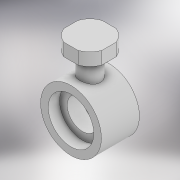
# Autodesk Inventor part: Sholder
Saved by Autodesk Inventor 2022 (Build 260153000, 153)
## iProperties
Created: 2022-02-25
Part Number: Sholder
Material: Generic
Document SubType Name: Modeling
Designer: joshw
Density: 1 g/cm^3
Appearance: Default
Author: joshw
Autodesk Inventor part; units mm, degrees
ref_plane "YZ Plane" through (0, 0, 0) normal (1, 0, 0) x (0, 1, 0)
ref_plane "XZ Plane" through (0, 0, 0) normal (0, 1, 0) x (-1, 0, 0)
ref_plane "XY Plane" through (0, 0, 0) normal (0, 0, 1) x (1, 0, 0)
sketch "Sketch1" plane through (0, 0, 0) normal (0, 0, 1) x (1, 0, 0)
  point P0 (0, 0)
sketch "Sketch2" plane through (0, 0, 0) normal (0, 0, 1) x (1, 0, 0)
  line L0 (12.1777, -1.5396) -> (4.6777, -1.5396) construction
  line L1 (4.6777, -1.5396) -> (4.6777, -5.5396) construction
  line L2 (4.6777, -5.5396) -> (12.1777, -5.5396) construction
  line L3 (12.1777, -5.5396) -> (12.1777, -1.5396) construction
  line L4 (8.4277, -4.7896) -> (12.4277, -4.7896)
  line L5 (12.4277, -4.7896) -> (12.4277, -2.2896)
  line L6 (12.4277, -2.2896) -> (8.4277, -2.2896)
  line L7 (8.4277, -2.2896) -> (8.4277, -4.7896)
  line L8 (8.4277, -2.2896) -> (8.4277, -8.9787)
  line L9 (8.4277, -8.9787) -> (10.4777, -8.9787)
  line L10 (10.4777, -8.9787) -> (10.4777, -4.7896)
  line L11 (9.1419, -2.2896) -> (9.1419, -1.5396) construction
  line L12 (9.1419, -4.7896) -> (9.1419, -5.5396) construction
  point P0 (0, 0)
  dimension "d0" = 7.5
  dimension "d1" = 4
  dimension "d2" = 8
  dimension "d3" = 2.5
  dimension "d4" = 4.1
  dimension "d6" = 0.75
  constraints: 26 end point, 6 perpendicular, 5 point on line, 4 parallel, 2 horizontal, 1 collinear, 1 vertical
  measures "d0" distance of L2.end L2.start
  measures "d1" distance of L2.start L1.start
  measures "d2" diameter of L5 L7
  measures "d3" distance between parallel lines of L6 L4
  measures "d4" diameter of L10 L7
  measures "d6" distance of L12.start L12.end
revolve "Revolution1" add sketch "Sketch2" angle 360 about axis through (8.4277, -2.2896, 0) along (0, -1, 0)
sketch "Sketch3" plane through (8.4277, -8.9787, 0) normal (0, -1, 0) x (1, 0, 0)
  line L0 (6, 3.75) -> (-6, 3.75)
  line L1 (-6, 3.75) -> (-6, -3.75)
  line L2 (-6, -3.75) -> (6, -3.75)
  line L3 (6, -3.75) -> (6, 3.75)
  line L4 (6, 3.75) -> (-6, -3.75) construction
  line L5 (-6, 3.75) -> (6, -3.75) construction
  circle A0 centre (0, 0) radius 2.05 projected
  point P0 (-8.4277, 0)
  point P1 (0, 0)
  dimension "d7" = 12
  dimension "d8" = 7.5
  constraints: 12 end point, 3 midpoint, 2 coincident, 2 parallel, 1 horizontal, 1 perpendicular
  measures "d7" distance of L2.end L1.end
  measures "d8" distance of L1.end L0.end
extrude "Extrusion1" add sketch "Sketch3" along normal blind 12 contours L3 L2 L1 L0 | A0
sketch "Sketch4" plane through (14.4277, -8.9787, -3.75) normal (0, 0, -1) x (-1, 0, 0)
  line L0 (12, 0) -> (0, 0) projected
  line L1 (0, 0) -> (0, -12) projected
  line L2 (12, -12) -> (0, -12) projected
  line L3 (12, 0) -> (12, -12) projected
  circle A0 centre (6, -6) radius 6
  point P0 (14.4277, 8.9787)
  point P1 (0, -6)
  point P2 (6, 0)
  point P3 (12, -6)
  point P4 (6, -12)
  constraints: 3 tangent, 1 centre point
extrude "Extrusion2" cut sketch "Sketch4" against normal blind 12 contours L3 A0 L0 | A0 L1 L0 | L3 L2 A0 | A0 L2 L1
sketch "Sketch6" plane through (0, 0, 0) normal (0, 0, 1) x (1, 0, 0)
  circle A0 centre (8.4277, -14.9787) radius 6 projected
  circle A1 centre (8.4277, -14.9787) radius 3
  point P0 (0, 0)
  dimension "d13" = 6
  constraints: 1 centre point, 1 coincident
  measures "d13" diameter of A1
extrude "Extrusion3" cut sketch "Sketch6" along normal mid plane 3 contours A1
sketch "Sketch7" plane through (8.4277, -14.9787, 1.5) normal (0, 0, -1) x (-1, 0, 0)
  circle A0 centre (0, 0) radius 3 projected
  circle A1 centre (0, 0) radius 4.5
  point P0 (8.4277, 14.9787)
  dimension "d16" = 9
  constraints: 1 centre point, 1 coincident
  measures "d16" diameter of A1
extrude "Extrusion4" cut sketch "Sketch7" against normal blind 8.25 contours A0 | A1
sketch "Sketch8" plane through (8.4277, -14.9787, -1.5) normal (0, 0, 1) x (1, 0, 0)
  circle A0 centre (0, 0) radius 4.5 projected
  point P0 (-8.4277, 14.9787)
extrude "Extrusion5" cut sketch "Sketch8" against normal blind 8.25
sketch "Sketch9" plane through (8.4277, -2.2896, 0) normal (0, 1, 0) x (1, 0, 0)
  circle A0 centre (0, 0) radius 4 projected
  line L0 (3.75, -3.75) -> (-3.75, -3.75)
  line L1 (-3.75, -3.75) -> (-3.75, 3.75)
  line L2 (-3.75, 3.75) -> (3.75, 3.75)
  line L3 (3.75, 3.75) -> (3.75, -3.75)
  line L4 (3.75, -3.75) -> (-3.75, 3.75) construction
  line L5 (-3.75, -3.75) -> (3.75, 3.75) construction
  point P0 (-3.75, -1.3919)
  point P1 (-3.75, 1.3919)
  point P2 (1.3919, -3.75)
  point P3 (-1.3919, -3.75)
  point P4 (3.75, 1.3919)
  point P5 (3.75, -1.3919)
  point P6 (-1.3919, 3.75)
  point P7 (1.3919, 3.75)
  dimension "d23" = 7.5
  constraints: 12 end point, 2 midpoint, 2 parallel, 2 perpendicular, 1 horizontal
  measures "d23" distance of L1.end L2.end
extrude "Extrusion6" cut sketch "Sketch9" against normal up to surface (2.5 mm away) contours A0 L3 | L2 A0 | A0 L0 | L1 A0
sketch "Sketch10" plane through (8.4277, -8.9787, 0) normal (0, -1, 0) x (1, 0, 0)
  line L0 (-1.3919, 3.75) -> (1.3919, 3.75) projected
  arc A0 (3.75, 1.3919) -> (1.3919, 3.75) centre (0, 0) ccw projected
  line L1 (3.75, 1.3919) -> (3.75, -1.3919) projected
  arc A1 (1.3919, -3.75) -> (3.75, -1.3919) centre (0, 0) ccw projected
  line L2 (1.3919, -3.75) -> (-1.3919, -3.75) projected
  arc A2 (-3.75, -1.3919) -> (-1.3919, -3.75) centre (0, 0) ccw projected
  line L3 (-3.75, -1.3919) -> (-3.75, 1.3919) projected
  arc A3 (-1.3919, 3.75) -> (-3.75, 1.3919) centre (0, 0) ccw projected
  circle A4 centre (0, 0) radius 2.05 projected
  point P0 (-8.4277, 0)
extrude "Extrusion7" add sketch "Sketch10" along normal up to surface contours A4 round surface about axis through (8.4277, -14.9787, -3.75) along (0, 0, 1) radius 6 far side no
body "Solid1"
